Autodesk Inventor part; units mm, degrees
(part 6 of 6)
sketch "Sketch33" plane through (-9.1776, 2.1219, -2.7) normal (0, 0, -1) x (-0.9998912, 0.0147508, 0)
  circle A0 centre (-4.4584, -2.0563) radius 3.95 projected
  line L0 (-4.4584, 2.3152) -> (-4.4584, -0.6077) construction
  arc A1 (-1.0545, -4.7993) -> (-0.0358, -5.127) centre (0.6426, -1.2701) ccw
  arc A2 (-0.0358, -5.127) -> (0.1719, -4.8036) centre (-4.4584, -2.0563) ccw
  arc A3 (-0.5493, -4.0131) -> (-0.4196, -3.7292) centre (-4.4584, -2.0563) ccw
  arc A4 (-0.4196, -3.7292) -> (0.6501, -3.7566) centre (0.2144, 0.1352) ccw
  arc A5 (0.6501, -3.7566) -> (0.7584, -3.3878) centre (-4.4584, -2.0563) ccw
  arc A6 (-0.1563, -2.8325) -> (-0.1119, -2.5236) centre (-4.4584, -2.0563) ccw
  arc A7 (0.7584, -3.3878) -> (-0.1563, -2.8325) centre (-1.7122, -6.4263) ccw
  arc A8 (0.1719, -4.8036) -> (-0.5493, -4.0131) centre (-3.0546, -7.023) ccw
  arc A9 (-0.5493, -0.0996) -> (0.1719, 0.691) centre (-3.0546, 2.9103) ccw
  arc A10 (0.1719, 0.691) -> (-0.0358, 1.0143) centre (-4.4584, -2.0563) ccw
  arc A11 (-0.0358, 1.0143) -> (-1.0545, 0.6866) centre (0.6426, -2.8426) ccw
  arc A12 (-1.0545, 0.6866) -> (-1.2589, 0.9225) centre (-4.4584, -2.0563) ccw
  arc A13 (-1.2589, 0.9225) -> (-0.7896, 1.8842) centre (-4.5107, 3.1046) ccw
  arc A14 (-0.7896, 1.8842) -> (-1.0801, 2.1359) centre (-4.4584, -2.0563) ccw
  arc A15 (-1.0801, 2.1359) -> (-1.9652, 1.5345) centre (0.6575, -1.3737) ccw
  arc A16 (-1.9652, 1.5345) -> (-2.2277, 1.7032) centre (-4.4584, -2.0563) ccw
  arc A17 (-5.5395, 2.1794) -> (-5.8389, 2.0915) centre (-4.4584, -2.0563) ccw
  arc A18 (-5.4143, 3.2421) -> (-5.5395, 2.1794) centre (-1.6241, 2.257) ccw
  arc A19 (-5.0339, 3.2968) -> (-5.4143, 3.2421) centre (-4.4584, -2.0563) ccw
  arc A20 (-4.6144, 2.3124) -> (-5.0339, 3.2968) centre (-8.393, 1.2838) ccw
  arc A21 (-4.3023, 2.3124) -> (-4.6144, 2.3124) centre (-4.4584, -2.0563) ccw
  arc A22 (-3.8828, 3.2968) -> (-4.3023, 2.3124) centre (-0.5237, 1.2838) ccw
  arc A23 (-3.5024, 3.2421) -> (-3.8828, 3.2968) centre (-4.4584, -2.0563) ccw
  arc A24 (-3.3773, 2.1794) -> (-3.5024, 3.2421) centre (-7.2926, 2.257) ccw
  arc A25 (-3.0779, 2.0915) -> (-3.3773, 2.1794) centre (-4.4584, -2.0563) ccw
  arc A26 (-2.398, 2.9178) -> (-3.0779, 2.0915) centre (0.2579, 0.04) ccw
  arc A27 (-2.2277, 1.7032) -> (-2.0484, 2.7582) centre (-5.9626, 2.8808) ccw
  arc A28 (-2.0484, 2.7582) -> (-2.398, 2.9178) centre (-4.4584, -2.0563) ccw
  arc A29 (-8.4971, -0.3834) -> (-9.5668, -0.3561) centre (-9.1312, -4.2479) ccw
  arc A30 (-9.5668, -0.3561) -> (-9.6751, -0.7248) centre (-4.4584, -2.0563) ccw
  arc A31 (-9.6751, -0.7248) -> (-8.7604, -1.2802) centre (-7.2046, 2.3136) ccw
  arc A32 (-8.7604, -1.2802) -> (-8.8048, -1.589) centre (-4.4584, -2.0563) ccw
  arc A33 (-8.8048, -1.589) -> (-9.8389, -1.8642) centre (-8.3245, -5.4756) ccw
  arc A34 (-9.8389, -1.8642) -> (-9.8389, -2.2485) centre (-4.4584, -2.0563) ccw
  arc A35 (-8.8048, -2.5236) -> (-8.7604, -2.8325) centre (-4.4584, -2.0563) ccw
  arc A36 (-9.8389, -2.2485) -> (-8.8048, -2.5236) centre (-8.3245, 1.3629) ccw
  arc A37 (-8.7604, -2.8325) -> (-9.6751, -3.3878) centre (-7.2046, -6.4263) ccw
  arc A38 (-9.5668, -3.7566) -> (-8.4971, -3.7292) centre (-9.1312, 0.1352) ccw
  arc A39 (-9.6751, -3.3878) -> (-9.5668, -3.7566) centre (-4.4584, -2.0563) ccw
  arc A40 (-6.8683, -6.8708) -> (-6.5187, -7.0305) centre (-4.4584, -2.0563) ccw
  arc A41 (-6.689, -5.8159) -> (-6.8683, -6.8708) centre (-2.9541, -6.9935) ccw
  arc A42 (-6.9515, -5.6472) -> (-6.689, -5.8159) centre (-4.4584, -2.0563) ccw
  arc A43 (-7.8367, -6.2485) -> (-6.9515, -5.6472) centre (-9.5742, -2.739) ccw
  arc A44 (-8.1271, -5.9969) -> (-7.8367, -6.2485) centre (-4.4584, -2.0563) ccw
  arc A45 (-7.8622, -4.7993) -> (-7.6578, -5.0352) centre (-4.4584, -2.0563) ccw
  arc A46 (-7.6578, -5.0352) -> (-8.1271, -5.9969) centre (-4.406, -7.2173) ccw
  arc A47 (-8.4971, -3.7292) -> (-8.3675, -4.0131) centre (-4.4584, -2.0563) ccw
  arc A48 (-9.0887, -4.8036) -> (-8.8809, -5.127) centre (-4.4584, -2.0563) ccw
  arc A49 (-8.3675, -4.0131) -> (-9.0887, -4.8036) centre (-5.8622, -7.023) ccw
  arc A50 (-8.8809, -5.127) -> (-7.8622, -4.7993) centre (-9.5593, -1.2701) ccw
  arc A51 (-0.4196, -0.3834) -> (-0.5493, -0.0996) centre (-4.4584, -2.0563) ccw
  arc A52 (0.6501, -0.3561) -> (-0.4196, -0.3834) centre (0.2144, -4.2479) ccw
  arc A53 (0.7584, -0.7248) -> (0.6501, -0.3561) centre (-4.4584, -2.0563) ccw
  arc A54 (-0.1119, -1.589) -> (-0.1563, -1.2802) centre (-4.4584, -2.0563) ccw
  arc A55 (-0.1563, -1.2802) -> (0.7584, -0.7248) centre (-1.7122, 2.3136) ccw
  arc A56 (0.9222, -2.2485) -> (0.9222, -1.8642) centre (-4.4584, -2.0563) ccw
  arc A57 (-0.1119, -2.5236) -> (0.9222, -2.2485) centre (-0.5923, 1.3629) ccw
  arc A58 (0.9222, -1.8642) -> (-0.1119, -1.589) centre (-0.5923, -5.4756) ccw
  arc A59 (-5.8389, 2.0915) -> (-6.5187, 2.9178) centre (-9.1747, 0.04) ccw
  arc A60 (-6.5187, 2.9178) -> (-6.8683, 2.7582) centre (-4.4584, -2.0563) ccw
  arc A61 (-6.8683, 2.7582) -> (-6.689, 1.7032) centre (-2.9541, 2.8808) ccw
  arc A62 (-6.5187, -7.0305) -> (-5.8389, -6.2041) centre (-9.1747, -4.1527) ccw
  arc A63 (-5.8389, -6.2041) -> (-5.5395, -6.292) centre (-4.4584, -2.0563) ccw
  arc A64 (-5.5395, -6.292) -> (-5.4143, -7.3548) centre (-1.6241, -6.3697) ccw
  arc A65 (-5.4143, -7.3548) -> (-5.0339, -7.4095) centre (-4.4584, -2.0563) ccw
  arc A66 (-4.6144, -6.4251) -> (-4.3023, -6.4251) centre (-4.4584, -2.0563) ccw
  arc A67 (-5.0339, -7.4095) -> (-4.6144, -6.4251) centre (-8.393, -5.3965) ccw
  arc A68 (-3.3773, -6.292) -> (-3.0779, -6.2041) centre (-4.4584, -2.0563) ccw
  arc A69 (-3.8828, -7.4095) -> (-3.5024, -7.3548) centre (-4.4584, -2.0563) ccw
  arc A70 (-3.5024, -7.3548) -> (-3.3773, -6.292) centre (-7.2926, -6.3697) ccw
  arc A71 (-4.3023, -6.4251) -> (-3.8828, -7.4095) centre (-0.5237, -5.3965) ccw
  arc A72 (-8.3675, -0.0996) -> (-8.4971, -0.3834) centre (-4.4584, -2.0563) ccw
  arc A73 (-9.0887, 0.691) -> (-8.3675, -0.0996) centre (-5.8622, 2.9103) ccw
  arc A74 (-8.8809, 1.0143) -> (-9.0887, 0.691) centre (-4.4584, -2.0563) ccw
  arc A75 (-7.8622, 0.6866) -> (-8.8809, 1.0143) centre (-9.5593, -2.8426) ccw
  arc A76 (-7.6578, 0.9225) -> (-7.8622, 0.6866) centre (-4.4584, -2.0563) ccw
  arc A77 (-6.689, 1.7032) -> (-6.9515, 1.5345) centre (-4.4584, -2.0563) ccw
  arc A78 (-7.8367, 2.1359) -> (-8.1271, 1.8842) centre (-4.4584, -2.0563) ccw
  arc A79 (-6.9515, 1.5345) -> (-7.8367, 2.1359) centre (-9.5742, -1.3737) ccw
  arc A80 (-8.1271, 1.8842) -> (-7.6578, 0.9225) centre (-4.406, 3.1046) ccw
  arc A81 (-1.2589, -5.0352) -> (-1.0545, -4.7993) centre (-4.4584, -2.0563) ccw
  arc A82 (-0.7896, -5.9969) -> (-1.2589, -5.0352) centre (-4.5107, -7.2173) ccw
  arc A83 (-1.0801, -6.2485) -> (-0.7896, -5.9969) centre (-4.4584, -2.0563) ccw
  arc A84 (-2.2277, -5.8159) -> (-1.9652, -5.6472) centre (-4.4584, -2.0563) ccw
  arc A85 (-1.9652, -5.6472) -> (-1.0801, -6.2485) centre (0.6575, -2.739) ccw
  arc A86 (-2.0484, -6.8708) -> (-2.2277, -5.8159) centre (-5.9626, -6.9935) ccw
  arc A87 (-3.0779, -6.2041) -> (-2.398, -7.0305) centre (0.2579, -4.1527) ccw
  arc A88 (-2.398, -7.0305) -> (-2.0484, -6.8708) centre (-4.4584, -2.0563) ccw
  point P0 (-9.2079, -1.9863)
  constraints: 2 end point, 1 vertical, 2 other
extrude "Extrusion29" add sketch "Sketch33" along normal blind 2.5
fillet "Fillet7" radius 0.2 1 edges at (-0.8004, -0.0583, -5.2)
fillet "Fillet8" radius 0.2 2 edges at (-2.4113, -4.8495, -3.95) (-2.7632, -5.004, -3.95)
fillet "Fillet8" radius 0.2 2 edges at (-3.4308, -4.1677, -3.95) (-3.7315, -4.2512, -3.95)
pattern_circular "Circular Pattern3" count 22 over 360 about axis through (-4.75, 0, -5.2) along (0, 0, 1) of "Fillet8"
body "Solid1"
